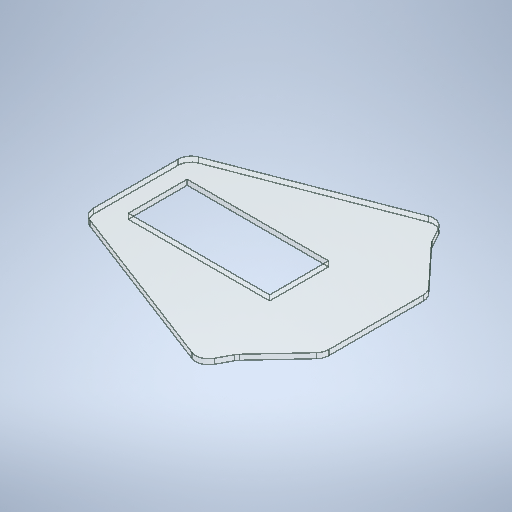
# Autodesk Inventor part: Screen Cover
Saved by Autodesk Inventor 2025 (Build 290162000, 162)
## iProperties
Created: 2025-04-19
Part Number: Screen Cover
Material: Generic
Document SubType Name: Modeling
Designer: User
Density: 1 g/cm^3
Appearance: Default
Author: User
Autodesk Inventor part; units mm, degrees
ref_plane "YZ Plane" through (0, 0, 0) normal (1, 0, 0) x (0, 1, 0)
ref_plane "XZ Plane" through (0, 0, 0) normal (0, 1, 0) x (-1, 0, 0)
ref_plane "XY Plane" through (0, 0, 0) normal (0, 0, 1) x (1, 0, 0)
sketch "Sketch1" plane through (0, 0, 0) normal (0, 1, 0) x (-1, 0, 0)
  line L0 (0, 0) -> (32.4, 0)
  line L1 (32.4, 0) -> (32.4, -13.5)
  line L2 (32.4, -13.5) -> (0, -13.5)
  line L3 (0, -13.5) -> (0, 0)
  line L4 (-5, 5) -> (37.4, 5)
  line L5 (37.4, 5) -> (37.4, -18.5)
  line L6 (37.4, -18.5) -> (-5, -18.5)
  line L7 (-5, -18.5) -> (-5, 5)
  line L8 (37.4, 5) -> (-5, 21.2758)
  line L9 (-5, 21.2758) -> (-5, -34.7758)
  line L10 (-5, -34.7758) -> (37.4, -18.5)
  line L11 (-5, 21.2758) -> (-8.0516, 15.5367)
  line L12 (-8.0516, 15.5367) -> (-17.644, 5.25)
  line L13 (-17.644, 5.25) -> (-17.644, -18.75)
  line L14 (-17.644, -18.75) -> (-8.0516, -29.0367)
  line L15 (-8.0516, -29.0367) -> (-5, -34.7758)
  point P0 (-5, -6.75)
  dimension "d0" = 32.4
  dimension "d1" = 13.5
  dimension "d2" = 5
  dimension "d5" = 21
  dimension "d6" = 21
  dimension "d8" = 28
  dimension "d9" = 28
  dimension "d11" = 6.5
  dimension "d12" = 24
  dimension "d13" = 6.5
  dimension "d15" = 165
  dimension "d16" = 165
  constraints: 32 end point, 4 parallel, 2 perpendicular, 2 vertical, 1 collinear, 1 horizontal, 1 midpoint, 3 other
  measures "d0" distance of L1.end L2.end
  measures "d1" distance of L0.end L1.end
  measures "d2" distance between parallel lines of L3 L7
  measures "d5" angle of L4 L8
  measures "d6" angle of L6 L10
  measures "d8" angle of L9 L11
  measures "d9" angle of L9 L15
  measures "d11" distance of L8.end L11.end
  measures "d12" distance of L12.end L13.end
  measures "d13" distance of L14.end L9.end
  measures "d15" angle of L11 L12
  measures "d16" angle of L15 L14
extrude "Extrusion1" add sketch "Sketch1" along normal blind 1.2
fillet "Fillet1" radius 3 8 edges at (5, 0.6, 21.2758) (17.644, 0.6, 5.25) (17.644, 0.6, -18.75) (5, 0.6, -34.7758) (8.0516, 0.6, -29.0367) (8.0516, 0.6, 15.5367) (-37.4, 0.6, 5) (-37.4, 0.6, -18.5)
equation "\"d6\" = d5"
equation "\"d9\" = d8"
equation "\"d13\" = d11"
equation "\"d16\" = d15"
body "Solid1"
